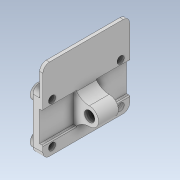
# Autodesk Inventor part: supCamnovo
Saved by Autodesk Inventor 2020.4 (Build 244396000, 396)
## iProperties
Created: 2021-09-09
Part Number: supCamnovo
Material: Generic
Document SubType Name: Modeling
Designer: becca
Density: 1 g/cm^3
Appearance: Default
Author: becca
Autodesk Inventor part; units mm, degrees
note: some values were not read from the file. Chosen so that the rebuilt part matches the saved one: edges of "Fillet2".
ref_plane "YZ Plane" through (0, 0, 0) normal (1, 0, 0) x (0, 1, 0)
ref_plane "XZ Plane" through (0, 0, 0) normal (0, 1, 0) x (-1, 0, 0)
ref_plane "XY Plane" through (0, 0, 0) normal (0, 0, 1) x (1, 0, 0)
sketch "Sketch3" plane through (0, 0, 0) normal (0, 0, 1) x (1, 0, 0)
  line L0 (26, 0) -> (26, 25)
  line L1 (26, 25) -> (2.3151, 25)
  circle A0 centre (2.2, 2.2) radius 2.2
  circle A1 centre (2.2, 2.2) radius 1.1
  circle A2 centre (2.2, 14.7) radius 1.1
  circle A3 centre (2.2, 14.7) radius 2.2
  circle A4 centre (23.2, 2.2) radius 2.2
  circle A5 centre (23.2, 2.2) radius 1.1
  circle A6 centre (23.2, 14.7) radius 1.1
  circle A7 centre (23.2, 14.7) radius 2.2
  line L2 (2.2, 2.2) -> (-0.6, 2.2)
  line L3 (-0.6, 2.2) -> (-0.6, 0)
  line L4 (-0.6, 0) -> (2.2, 0)
  line L5 (2.2, 0) -> (2.2, 2.2)
  line L6 (-0.6, 0) -> (26, 0)
  line L7 (26, 0) -> (26, 25)
  line L8 (26, 25) -> (-0.6, 25)
  line L9 (-0.6, 25) -> (-0.6, 0)
  line L10 (-0.6, 25) -> (26, 25)
  line L11 (26, 25) -> (26, 18)
  line L12 (26, 18) -> (-0.6, 18)
  line L13 (-0.6, 18) -> (-0.6, 25)
  point P0 (0, 0)
  point P1 (-0.6, 18)
  dimension "d14" = 25
  dimension "d15" = 4.4
  dimension "d16" = 2.2
  dimension "d18" = 2.2
  dimension "d19" = 4.4
  dimension "d21" = 4.4
  dimension "d22" = 2.2
  dimension "d23" = 4.4
  dimension "d25" = 7
  constraints: 28 end point, 8 centre point, 6 parallel, 4 coincident, 3 horizontal, 3 perpendicular, 1 point on line
  measures "d14" distance of L0.end L0.start
  measures "d15" diameter of A0
  measures "d16" diameter of A1
  measures "d18" diameter of A2
  measures "d19" diameter of A3
  measures "d21" diameter of A4
  measures "d22" diameter of A5
  measures "d23" diameter of A7
  measures "d25" distance of L10.end L11.end
extrude "Extrusion1" add sketch "Sketch3" along normal blind 3 contours A4 | L6 A0 L2 L9 L12 L0 | L5 A1 L2 A0 | L4 L3 L2 A0 | A0 L2 A1 L5 | A3 | A7
sketch "Sketch5" plane through (0, 0, 3) normal (0, 0, 1) x (1, 0, 0)
  line L0 (26, 0) -> (26, 25)
  line L1 (26, 25) -> (2.3151, 25)
  circle A0 centre (2.2, 2.2) radius 2.2
  circle A1 centre (2.2, 2.2) radius 1.1
  circle A2 centre (2.2, 14.7) radius 1.1
  circle A3 centre (2.2, 14.7) radius 2.2
  circle A4 centre (23.2, 2.2) radius 2.2
  circle A5 centre (23.2, 2.2) radius 1.1
  circle A6 centre (23.2, 14.7) radius 1.1
  circle A7 centre (23.2, 14.7) radius 2.2
  line L2 (2.2, 2.2) -> (-0.6, 2.2)
  line L3 (-0.6, 2.2) -> (-0.6, 0)
  line L4 (-0.6, 0) -> (2.2, 0)
  line L5 (2.2, 0) -> (2.2, 2.2)
  line L6 (-0.6, 0) -> (26, 0)
  line L7 (26, 0) -> (26, 25)
  line L8 (26, 25) -> (-0.6, 25)
  line L9 (-0.6, 25) -> (-0.6, 0)
  line L10 (-0.6, 25) -> (26, 25)
  line L11 (26, 25) -> (26, 18)
  line L12 (26, 18) -> (-0.6, 18)
  line L13 (-0.6, 18) -> (-0.6, 25)
  point P0 (0, 0)
  point P1 (0, 0)
  point P2 (-0.6, 18)
  point P3 (-0.6, 18)
  dimension "d28" = 25
  dimension "d29" = 4.4
  dimension "d30" = 2.2
  dimension "d31" = 2.2
  dimension "d32" = 4.4
  dimension "d33" = 4.4
  dimension "d34" = 2.2
  dimension "d35" = 4.4
  dimension "d36" = 7
  constraints: 28 end point, 8 centre point, 6 parallel, 4 coincident, 3 horizontal, 3 perpendicular, 1 point on line
  measures "d28" distance of L0.end L0.start
  measures "d29" diameter of A0
  measures "d30" diameter of A1
  measures "d31" diameter of A2
  measures "d32" diameter of A3
  measures "d33" diameter of A4
  measures "d34" diameter of A5
  measures "d35" diameter of A7
  measures "d36" distance of L10.end L11.end
extrude "Extrusion2" add sketch "Sketch5" against normal blind 1 contours L12 L9 L8 L1 L0
sketch "Sketch6" plane through (0, 0, 3) normal (0, 0, 1) x (1, 0, 0)
  line L0 (26, 0) -> (26, 25)
  line L1 (26, 25) -> (2.3151, 25)
  circle A0 centre (2.2, 2.2) radius 2.2
  circle A1 centre (2.2, 2.2) radius 1.1
  circle A2 centre (2.2, 14.7) radius 1.1
  circle A3 centre (2.2, 14.7) radius 2.2
  circle A4 centre (23.2, 2.2) radius 2.2
  circle A5 centre (23.2, 2.2) radius 1.1
  circle A6 centre (23.2, 14.7) radius 1.1
  circle A7 centre (23.2, 14.7) radius 2.2
  line L2 (2.2, 2.2) -> (-0.6, 2.2)
  line L3 (-0.6, 2.2) -> (-0.6, 0)
  line L4 (-0.6, 0) -> (2.2, 0)
  line L5 (2.2, 0) -> (2.2, 2.2)
  line L6 (-0.6, 0) -> (26, 0)
  line L7 (26, 0) -> (26, 25)
  line L8 (26, 25) -> (-0.6, 25)
  line L9 (-0.6, 25) -> (-0.6, 0)
  line L10 (-0.6, 25) -> (26, 25)
  line L11 (26, 25) -> (26, 18)
  line L12 (26, 18) -> (-0.6, 18)
  line L13 (-0.6, 18) -> (-0.6, 25)
  point P0 (0, 0)
  point P1 (0, 0)
  point P2 (-0.6, 18)
  dimension "d39" = 25
  dimension "d40" = 4.4
  dimension "d41" = 2.2
  dimension "d42" = 2.2
  dimension "d43" = 4.4
  dimension "d44" = 4.4
  dimension "d45" = 2.2
  dimension "d46" = 4.4
  dimension "d47" = 7
  constraints: 28 end point, 8 centre point, 6 parallel, 4 coincident, 3 horizontal, 3 perpendicular, 1 point on line
  measures "d39" distance of L0.end L0.start
  measures "d40" diameter of A0
  measures "d41" diameter of A1
  measures "d42" diameter of A2
  measures "d43" diameter of A3
  measures "d44" diameter of A4
  measures "d45" diameter of A5
  measures "d46" diameter of A7
  measures "d47" distance of L10.end L11.end
extrude "Extrusion3" add sketch "Sketch6" against normal blind 4.5 contours A4 | L5 A1 L2 A0 | A0 L2 A1 L5 | A3 | A7
fillet "Fillet1" radius 2 6 edges at (26, 25, 2.5) (-0.6, 25, 2.5) (26, 18, 1) (-0.6, 18, 1) (-0.6, 0, 1.5) (26, 0, 1.5)
thread "Thread1" size "M2.2x0.45" class "6H" standard "ANSI Metric M Profile" full length
thread "Thread2" size "M2.2x0.45" class "6H" standard "ANSI Metric M Profile" full length
thread "Thread3" size "M2.2x0.45" class "6H" standard "ANSI Metric M Profile" full length
thread "Thread4" size "M2.2x0.45" class "6H" standard "ANSI Metric M Profile" full length
sketch "Sketch7" plane through (0, 0, 3) normal (0, 0, 1) x (1, 0, 0)
  circle A0 centre (2.2, 2.2) radius 1.1 projected
  circle A1 centre (23.2, 14.7) radius 1.1 projected
  circle A2 centre (2.2, 2.2) radius 2.2 projected
  circle A3 centre (23.2, 14.7) radius 2.2 projected
  line L0 (-0.6, 3.85) -> (26, 3.85)
  line L1 (26, 3.85) -> (26, 13.05)
  line L2 (26, 13.05) -> (-0.6, 13.05)
  line L3 (-0.6, 13.05) -> (-0.6, 3.85)
  point P0 (0, 0)
  point P1 (23.2, 13.05)
  point P2 (2.2, 3.85)
  constraints: 8 end point, 2 parallel, 1 horizontal, 1 perpendicular
extrude "Extrusion4" cut sketch "Sketch7" against normal blind 1 contours L0 A2 | A2 L0 L3 L2 A3 L1 | A3 L2 picked at (2.5398, 3.9498) picked at (23.5398, 12.9502)
sketch "Sketch8" plane through (0, 0, 2) normal (0, 0, 1) x (1, 0, 0)
  line L0 (-0.6, 3.85) -> (-0.6, 13.05) projected
  line L1 (-0.6, 13.05) -> (26, 13.05) projected
  line L2 (-0.6, 3.85) -> (26, 3.85)
  line L3 (26, 3.85) -> (26, 13.05)
  line L4 (26, 13.05) -> (-0.6, 13.05)
  line L5 (-0.6, 13.05) -> (-0.6, 3.85)
  line L6 (26, 3.85) -> (-0.6, 3.85) projected
  line L7 (12.7, 3.85) -> (14.9828, 3.85)
  line L8 (14.9828, 3.85) -> (12.7, 3.85)
  line L9 (15.7821, 13.05) -> (15.7821, 3.85)
  line L10 (9.7, 3.85) -> (9.7, 13.05)
  point P0 (0, 0)
  point P1 (15.7821, 3.85)
  constraints: 16 end point, 5 point on line, 3 equal length, 3 perpendicular, 1 horizontal, 1 midpoint
extrude "Extrusion5" add sketch "Sketch8" along normal blind 10 contours L10 L1 L9 L2
fillet "Fillet2" radius 0.3 4 edges at (4.55, 13.05, 3) (4.55, 3.85, 3) (20.8911, 13.05, 3) (20.8911, 3.85, 3)
sketch "Sketch9" plane through (15.7821, 3.85, 2) normal (1, 0, 0) x (0, 0, -1)
  line L0 (0, 0) -> (0, 4.6)
  line L1 (-10, 0) -> (-10, 9.2) projected
  circle A0 centre (-5, 4.6) radius 1.6
  circle A1 centre (-5, 4.6) radius 2.75
  line L2 (-1, 0) -> (-5, 1.85)
  line L3 (-1, 9.2) -> (-10, 9.2) projected
  line L4 (-1, 9.2) -> (-5, 7.35)
  line L5 (0, 0) -> (-0.7, 0) projected
  line L6 (-10, 0) -> (0, 0)
  line L7 (0, 0) -> (0, 9.2)
  line L8 (0, 9.2) -> (-1, 9.2)
  line L9 (-0.7, 9.2) -> (0, 9.2) projected
  line L10 (-1, 0) -> (-1, -0.3) projected
  arc A2 (-1, 0) -> (-5, 1.85) centre (-4.8841, -3.1487) ccw
  arc A3 (-5, 7.35) -> (-1, 9.2) centre (-4.8841, 12.3487) ccw
  point P0 (2, -3.85)
  point P1 (-4.9177, 7.3488)
  point P2 (-4.9177, 1.8512)
  dimension "d69" = 3.2
  dimension "d70" = 5.5
  dimension "d73" = 5
  dimension "d74" = 5
  constraints: 12 end point, 6 point on circle, 4 centre point, 2 collinear, 1 coincident, 1 parallel, 1 perpendicular
  measures "d69" diameter of A0
  measures "d70" diameter of A1
  measures "d73" radius of A2
  measures "d74" radius of A3
extrude "Extrusion6" cut sketch "Sketch9" against normal blind 10 contours L6 L1 L3 L4 A1 L2 | L2 A2 | A3 L4
sketch "Sketch10" plane through (15.7821, 3.85, 2) normal (1, 0, 0) x (0, 0, -1)
  line L0 (0, 0) -> (0, 4.6)
  line L1 (-10, 0) -> (-10, 9.2)
  circle A0 centre (-5, 4.6) radius 1.6
  circle A1 centre (-5, 4.6) radius 2.75
  line L2 (-1, 0) -> (-5, 1.85)
  line L3 (-1, 9.2) -> (-10, 9.2)
  line L4 (-1, 9.2) -> (-5, 7.35)
  line L5 (0, 0) -> (-0.7, 0)
  line L6 (-10, 0) -> (0, 0)
  line L7 (0, 0) -> (0, 9.2)
  line L8 (0, 9.2) -> (-1, 9.2)
  line L9 (-0.7, 9.2) -> (0, 9.2)
  line L10 (-1, 0) -> (-1, -0.3)
  arc A2 (-1, 0) -> (-5, 1.85) centre (-4.8841, -3.1487) ccw
  arc A3 (-5, 7.35) -> (-1, 9.2) centre (-4.8841, 12.3487) ccw
  point P0 (2, -3.85)
  point P1 (2, -3.85)
  point P2 (-4.9177, 7.3488)
  point P3 (-4.9177, 1.8512)
  dimension "d75" = 3.2
  dimension "d76" = 5.5
  dimension "d77" = 5
  dimension "d78" = 5
  constraints: 22 end point, 6 point on circle, 4 centre point, 2 collinear, 1 coincident, 1 parallel, 1 perpendicular
  measures "d75" diameter of A0
  measures "d76" diameter of A1
  measures "d77" radius of A2
  measures "d78" radius of A3
extrude "Extrusion7" cut sketch "Sketch10" against normal blind 10 contours A0
thread "Thread5" size "M3.5x0.6" class "6H" standard "ANSI Metric M Profile" full length
body "Solid1"
